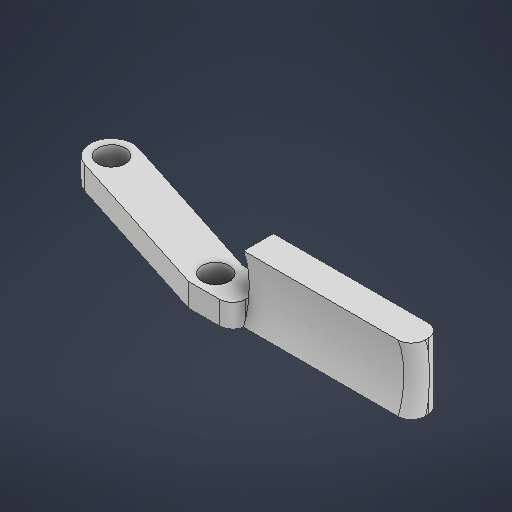
# Autodesk Inventor part: grips
Saved by Autodesk Inventor 2026.2 (Build 302298000, 298)
## iProperties
Created: 2026-04-07
Part Number: grips
Material: Generic
Document SubType Name: Modeling
Designer: Brian Wang
Density: 1 g/cm^3
Appearance: Default
Author: Brian Wang
Autodesk Inventor part; units mm, degrees
ref_plane "YZ Plane" through (0, 0, 0) normal (1, 0, 0) x (0, 1, 0)
ref_plane "XZ Plane" through (0, 0, 0) normal (0, 1, 0) x (-1, 0, 0)
ref_plane "XY Plane" through (0, 0, 0) normal (0, 0, 1) x (1, 0, 0)
sketch "Sketch1" plane through (0, 0, 0) normal (0, 1, 0) x (-1, 0, 0)
  line L0 (27.1998, -28.5532) -> (-70.2595, -28.5532)
  circle A0 centre (9.562, -47.3358) radius 2.075
  arc A1 (8.5638, -50.4287) -> (10.5601, -44.2429) centre (9.562, -47.3358) ccw
  circle A2 centre (-13.677, -39.8358) radius 2.075
  line L1 (10.5601, -44.2429) -> (-12.6789, -36.7429)
  line L2 (8.5638, -50.4287) -> (-14.6752, -42.9287)
  line L3 (-14.6752, -42.9287) -> (-44.6752, -42.9287)
  line L4 (-12.6789, -36.7429) -> (-19.3171, -36.7429)
  line L5 (-44.6752, -38.4058) -> (-44.6752, -42.9287)
  line L6 (-19.3171, -36.7429) -> (-44.6752, -38.4058)
  constraints: 14 end point, 3 centre point, 2 point on circle, 1 coincident, 1 horizontal
extrude "Extrusion1" add sketch "Sketch1" along normal blind 3.5
sketch "Sketch2" plane through (0, 3.5, 0) normal (0, 1, 0) x (1, 0, 0)
  line L0 (19.3171, 36.7429) -> (44.6752, 38.4058) projected
  line L1 (19.3171, 36.7429) -> (44.6752, 38.4058)
  line L2 (19.3171, 36.7429) -> (19.3171, 42.9287)
  line L3 (44.6752, 42.9287) -> (14.6752, 42.9287) projected
  line L4 (19.3171, 42.9287) -> (44.6752, 42.9287)
  line L5 (44.6752, 42.9287) -> (44.6752, 38.4058)
  point P0 (0, 0)
  point P1 (44.6752, 18.7005)
  point P2 (19.3171, 20.3635)
  point P3 (44.6752, 14.1776)
  constraints: 8 end point, 2 collinear, 1 perpendicular, 1 point on line, 1 vertical
extrude "Extrusion2" add sketch "Sketch2" along normal blind 6.5
sketch "Sketch3" plane through (44.6752, 0, -38.4058) normal (1, 0, 0) x (0, 0, -1)
  arc A0 (-19.7053, 10) -> (-19.7053, 0) centre (-5.5631, 5) ccw
  arc A1 (0, 0) -> (0, 10) centre (-14.1421, 5) ccw
  line L0 (-19.7053, 10) -> (-19.7053, 0)
  line L1 (0, 10) -> (0, 0)
  line L2 (4.5229, 10) -> (-1.6629, 10) projected
  line L3 (-19.7053, 10) -> (0, 10)
  line L4 (-24.2282, 0) -> (-19.7053, 0) projected
  line L5 (-1.6629, 0) -> (0, 0) projected
  line L6 (-19.7053, 0) -> (0, 0)
  point P0 (-38.4058, 0)
  dimension "d17" = 15
  dimension "d18" = 15
  constraints: 8 end point, 4 point on circle, 2 centre point, 1 collinear, 1 horizontal, 1 perpendicular
  measures "d17" radius of A0
  measures "d18" radius of A1
extrude "Extrusion3" cut sketch "Sketch3" against normal up to surface (25.3581 mm away)
fillet "Fillet1" radius 2 1 edges at (19.3171, 1.75, -36.7429)
fillet "Fillet3" radius 2 2 edges at (44.6752, 5, -39.2637) (44.6752, 5, -42.9287)
body "Solid1"
